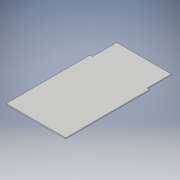
# Autodesk Inventor part: 89x49mm-PCB
Saved by Autodesk Inventor 2018 (Build 220112000, 112)
## iProperties
Created: 2018-04-06
Part Number: 89x49mm-PCB
Material: Generic
Document SubType Name: Modeling
Designer: bbramman
Density: 1 g/cm^3
Appearance: Default
Author: bbramman
Autodesk Inventor part; units mm, degrees
ref_plane "YZ Plane" through (0, 0, 0) normal (1, 0, 0) x (0, 1, 0)
ref_plane "XZ Plane" through (0, 0, 0) normal (0, 1, 0) x (-1, 0, 0)
ref_plane "XY Plane" through (0, 0, 0) normal (0, 0, 1) x (1, 0, 0)
sketch "Sketch1" plane through (0, 0, 0) normal (0, 1, 0) x (-1, 0, 0)
  line L0 (-24.5, 34.5) -> (24.5, 34.5)
  line L1 (24.5, 34.5) -> (24.5, -34.5)
  line L2 (-24.5, -34.5) -> (-24.5, 34.5)
  line L3 (-24.5, 34.5) -> (24.5, -34.5) construction
  line L4 (24.5, 34.5) -> (-24.5, -34.5) construction
  line L5 (22.5, -54.5) -> (-22.5, -54.5)
  line L6 (-22.5, -14.5) -> (22.5, -54.5) construction
  line L7 (22.5, -14.5) -> (-22.5, -54.5) construction
  line L8 (-22.5, -34.5) -> (-22.5, -54.5)
  line L9 (-22.5, -54.5) -> (22.5, -54.5)
  line L10 (22.5, -54.5) -> (22.5, -34.5)
  line L11 (22.5, -34.5) -> (24.5, -34.5)
  line L12 (-24.5, -34.5) -> (-22.5, -34.5)
  point P0 (0, 0)
  point P1 (0, -34.5)
  dimension "d0" = 49
  dimension "d1" = 69
  dimension "d2" = 45
  dimension "d3" = 40
  constraints: 26 end point, 4 midpoint, 2 horizontal, 2 parallel, 2 perpendicular
  measures "d0" distance of L1.end L2.start
  measures "d1" distance of L0.end L1.end
  measures "d2" distance of L5.start L5.end
  measures "d3" distance of L7.start L5.start
extrude "Extrusion1" add sketch "Sketch1" along normal mid plane 0.7874
body "Solid1"
